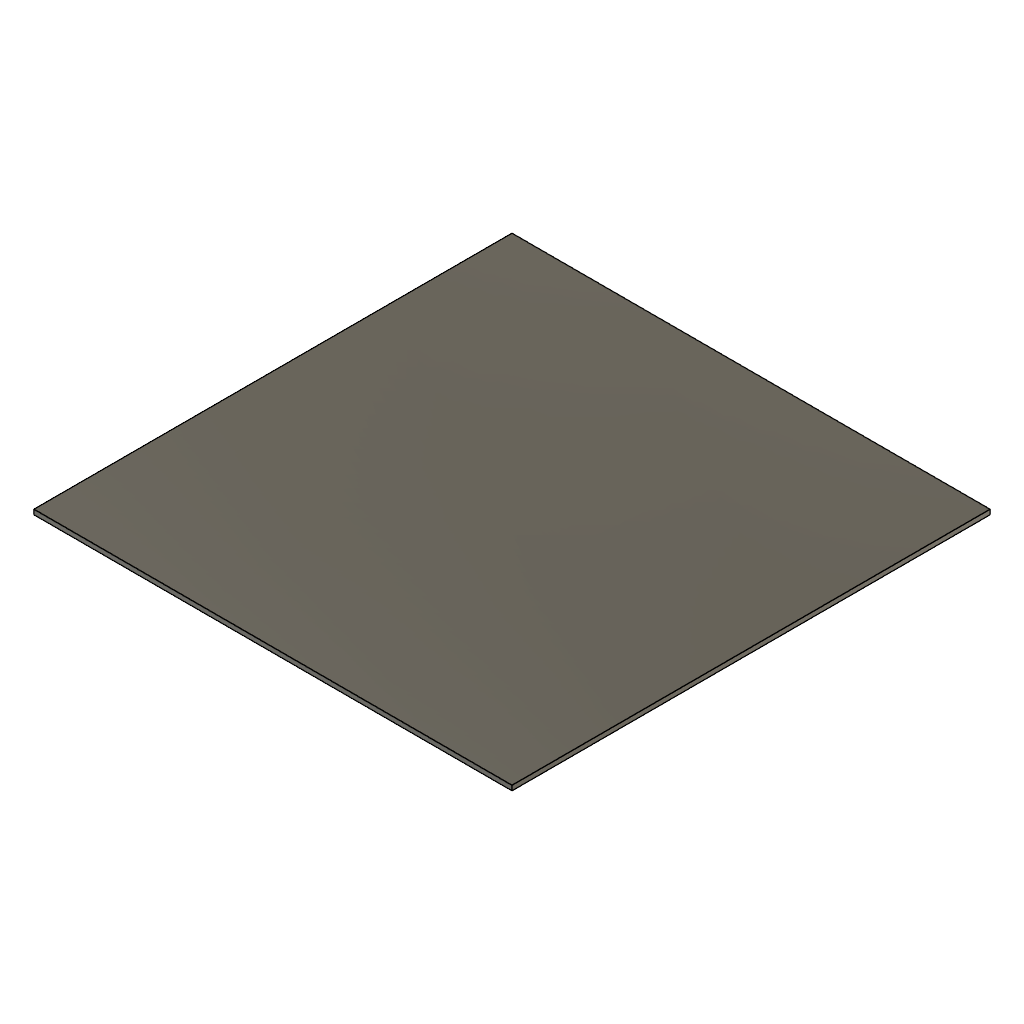
Assemblage (Autodesk Fusion 360 archive; units mm, degrees)
design "fond_plat"
part number: 2026-09-20-12-03-06-887
Autodesk Fusion 360 part; units mm, degrees
sketch "Esquisse1" plane through (0, 0, 0) normal (0, 0, 1) x (1, 0, 0)
  line L0 (-37.2128, 57.6344) -> (942.7872, 57.6344)
  line L1 (942.7872, 57.6344) -> (942.7872, -922.3656)
  line L2 (942.7872, -922.3656) -> (-37.2128, -922.3656)
  line L3 (-37.2128, -922.3656) -> (-37.2128, 57.6344)
  dimension "d1" = 980
  dimension "d2" = 980
  constraint horizontal L0
  constraint vertical L1
  constraint horizontal L2
  constraint vertical L3
  measures "d1" distance of L0.start L2.end
  measures "d2" distance of L0.start L0.end
extrude "Extrusion1" add sketch "Esquisse1" along normal blind 10
equation "d1 = 1000 mm - 10 mm - 10 mm"
equation "d2 = 1000 mm - 10 mm - 10 mm"

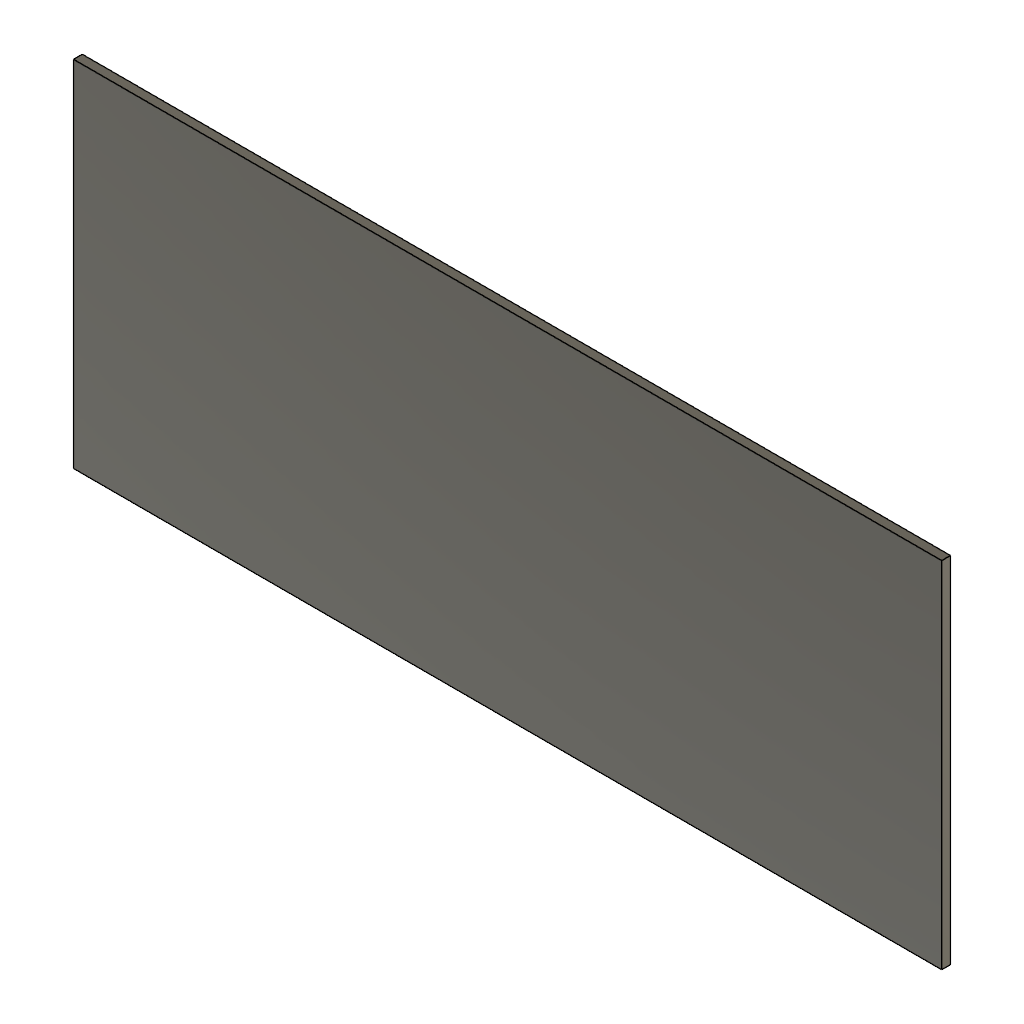
design "fond_droit"
part number: 2026-09-20-11-51-00-989
Autodesk Fusion 360 part; units mm, degrees
sketch "Esquisse1" plane through (0, 0, 0) normal (0, 1, 0) x (1, 0, 0)
  line L0 (-100, -60) -> (880, -60)
  line L1 (880, -60) -> (880, 340)
  line L2 (880, 340) -> (-100, 340)
  line L3 (-100, 340) -> (-100, -60)
  dimension "d1" = 980
  dimension "d2" = 400
  constraint horizontal L0
  constraint vertical L1
  constraint horizontal L2
  constraint vertical L3
  measures "d1" distance of L0.start L0.end
  measures "d2" distance of L0.start L2.end
extrude "Extrusion1" add sketch "Esquisse1" along normal blind 10
equation "d1 = 1000 mm - 10 mm - 10 mm"

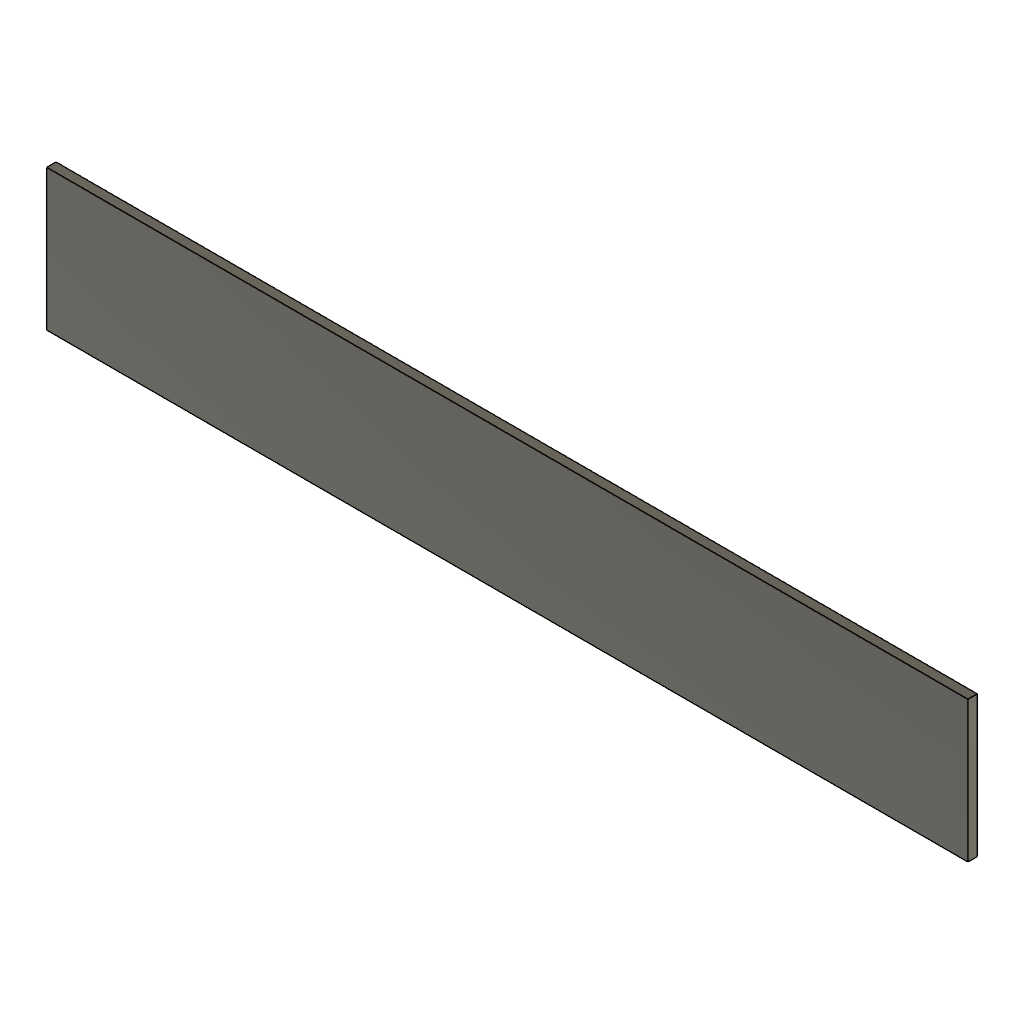
design "avant"
part number: 2026-09-20-11-55-13-038
Autodesk Fusion 360 part; units mm, degrees
sketch "Esquisse1" plane through (0, 0, 0) normal (0, 1, 0) x (1, 0, 0)
  line L0 (-33.9159, -73.41) -> (946.0841, -73.41)
  line L1 (946.0841, -73.41) -> (946.0841, 76.59)
  line L2 (946.0841, 76.59) -> (-33.9159, 76.59)
  line L3 (-33.9159, 76.59) -> (-33.9159, -73.41)
  dimension "d1" = 980
  dimension "d2" = 150
  constraint horizontal L0
  constraint vertical L1
  constraint horizontal L2
  constraint vertical L3
  measures "d1" distance of L0.start L0.end
  measures "d2" distance of L0.start L2.end
extrude "Extrusion1" add sketch "Esquisse1" along normal blind 10
equation "d1 = 1000 mm - 10 mm - 10 mm"

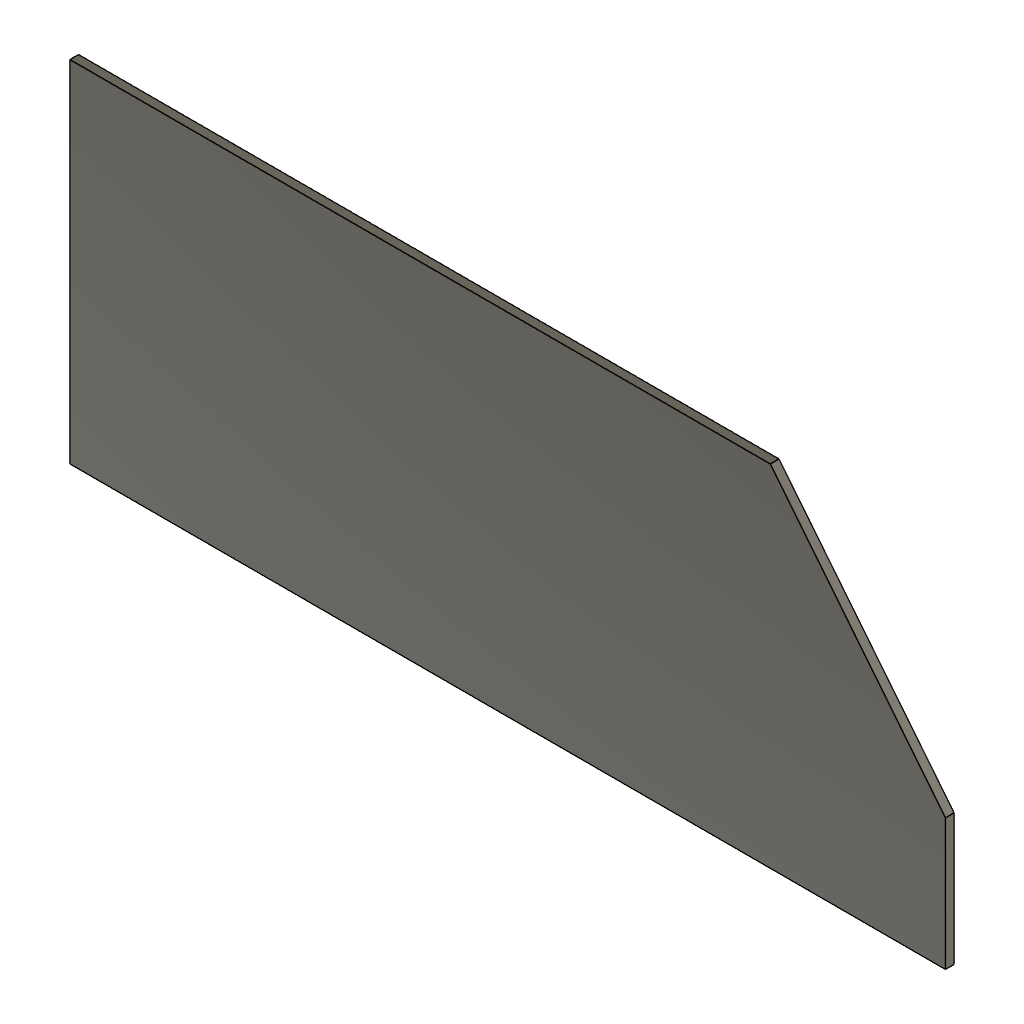
design "plaque_droite"
part number: 2026-09-20-11-41-58-876
Autodesk Fusion 360 part; units mm, degrees
sketch "Esquisse1" plane through (0, 0, 0) normal (0, 1, 0) x (1, 0, 0)
  line L0 (-23.5902, -87.415) -> (776.4098, -87.415)
  line L1 (976.4098, 162.585) -> (976.4098, 312.585)
  line L2 (976.4098, 312.585) -> (-23.5902, 312.585)
  line L3 (-23.5902, 312.585) -> (-23.5902, -87.415)
  line L4 (976.4098, 162.585) -> (776.4098, -87.415)
  dimension "d2" = 400
  dimension "d3" = 200
  dimension "d4" = 150
  dimension "d5" = 1000
  constraint horizontal L0
  constraint vertical L1
  constraint horizontal L2
  constraint vertical L3
  measures "d2" distance of L0.start L2.end
  measures "d3" distance of L1 L0.end
  measures "d4" distance of L1.end L1.start
  measures "d5" distance of L1.end L2.end
extrude "Extrusion1" add sketch "Esquisse1" along normal blind 10

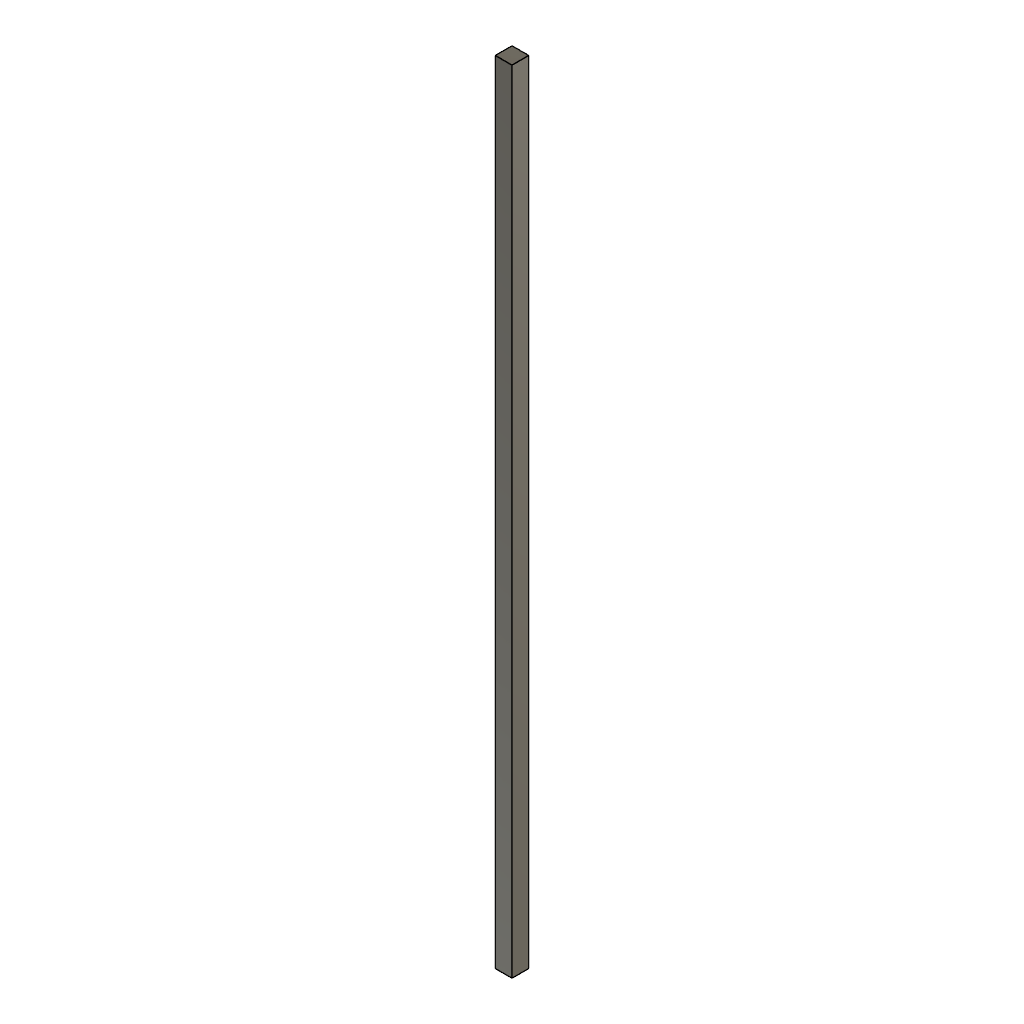
design "chevron940"
part number: 2026-09-20-12-08-54-033
Autodesk Fusion 360 part; units mm, degrees
sketch "Esquisse1" plane through (0, 0, 0) normal (0, 0, 1) x (1, 0, 0)
  line L0 (-61.9457, 47.4236) -> (-41.9457, 47.4236)
  line L1 (-41.9457, 47.4236) -> (-41.9457, 27.4236)
  line L2 (-41.9457, 27.4236) -> (-61.9457, 27.4236)
  line L3 (-61.9457, 27.4236) -> (-61.9457, 47.4236)
  dimension "d1" = 20
  dimension "d2" = 20
  constraint horizontal L0
  constraint vertical L1
  constraint horizontal L2
  constraint vertical L3
  measures "d1" distance of L0.start L2.end
  measures "d2" distance of L0.start L0.end
extrude "Extrusion1" add sketch "Esquisse1" along normal blind 940

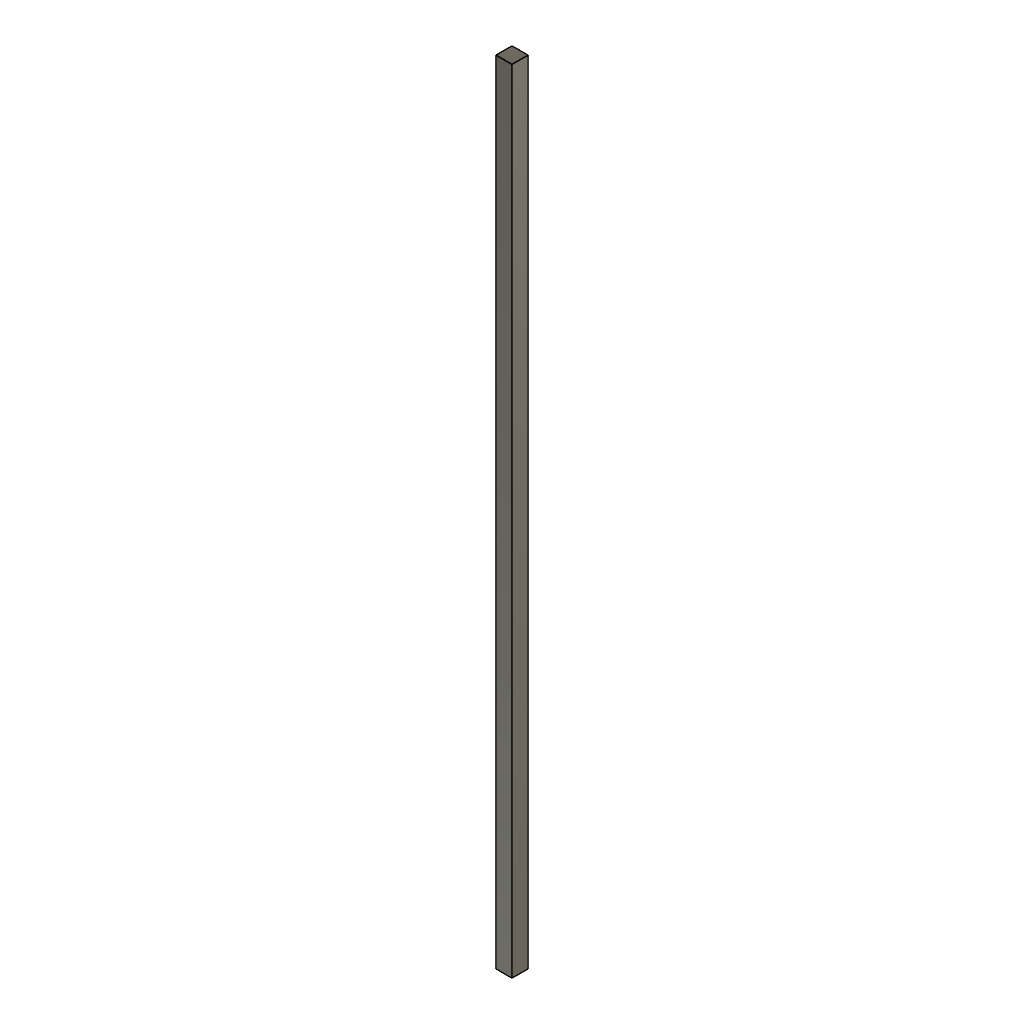
design "chevron980"
part number: 2026-09-20-12-08-54-033
Autodesk Fusion 360 part; units mm, degrees
sketch "Esquisse1" plane through (0, 0, 0) normal (0, 0, 1) x (1, 0, 0)
  line L0 (-61.9457, 47.4236) -> (-41.9457, 47.4236)
  line L1 (-41.9457, 47.4236) -> (-41.9457, 27.4236)
  line L2 (-41.9457, 27.4236) -> (-61.9457, 27.4236)
  line L3 (-61.9457, 27.4236) -> (-61.9457, 47.4236)
  dimension "d1" = 20
  dimension "d2" = 20
  constraint horizontal L0
  constraint vertical L1
  constraint horizontal L2
  constraint vertical L3
  measures "d1" distance of L0.start L2.end
  measures "d2" distance of L0.start L0.end
extrude "Extrusion1" add sketch "Esquisse1" along normal blind 980
